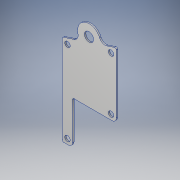
# Autodesk Inventor part: Column Plate
Saved by Autodesk Inventor 2019.4 (Build 234330000, 330)
## iProperties
Created: 2020-01-18
Part Number: Column Plate
Material: Aluminum 6061
Document SubType Name: Modeling
Designer: admin
Density: 2.7 g/cm^3
Appearance: Aluminum - Flat
Author: admin
Autodesk Inventor part; units mm, degrees
ref_plane "YZ Plane" through (0, 0, 0) normal (1, 0, 0) x (0, 1, 0)
ref_plane "XZ Plane" through (0, 0, 0) normal (0, 1, 0) x (-1, 0, 0)
ref_plane "XY Plane" through (0, 0, 0) normal (0, 0, 1) x (1, 0, 0)
sketch "Sketch1" plane through (0, 0, 0) normal (0, 0, 1) x (1, 0, 0)
  line L0 (0, 0) -> (-188.4, 0)
  line L1 (-188.4, 0) -> (-188.4, 316.0385)
  line L2 (-188.4, 316.0385) -> (0, 377.8495)
  circle A0 centre (-170.4, 303) radius 9.5
  circle A1 centre (-18, 353) radius 9.5
  circle A2 centre (-170.4, 18) radius 9.5
  circle A3 centre (-79, 86.5538) radius 88.9 construction
  line L3 (-188.4, 0) -> (-152.4, 0)
  line L4 (-152.4, 0) -> (-152.4, 150)
  line L5 (-152.4, 150) -> (0, 150)
  line L6 (0, 150) -> (0, 377.8495)
  circle A4 centre (-18, 168) radius 9.5
  circle A5 centre (-94.2, 287.3576) radius 88.9 construction
  circle A6 centre (-95, 363.5206) radius 16
  circle A7 centre (-95, 363.5206) radius 40
  dimension "d22" = 19
  dimension "d23" = 19
  dimension "d24" = 18
  dimension "d25" = 18
  dimension "d27" = 18
  dimension "d28" = 19
  dimension "d29" = 18
  dimension "d30" = 18
  dimension "d35" = 177.8
  dimension "d36" = 18
  dimension "d37" = 150
  dimension "d38" = 19
  dimension "d39" = 18
  dimension "d40" = 18
  dimension "d41" = 152.4
  dimension "d42" = 18
  dimension "d43" = 50
  dimension "d44" = 0
  dimension "d45" = 177.8
  dimension "d46" = 135
  dimension "d51" = 32
  dimension "d52" = 80
  dimension "d53" = 95
  constraints: 14 end point, 8 centre point, 2 point on line, 1 coincident, 1 horizontal, 1 parallel, 1 perpendicular, 1 tangent, 1 vertical
  measures "d22" diameter of A0
  measures "d23" diameter of A1
  measures "d24" distance from line of L1 A0.centre
  measures "d25" distance from line of L2 A0.centre
  measures "d27" distance from line of L2 A1.centre
  measures "d28" diameter of A2
  measures "d29" distance from line of L1 A2.centre
  measures "d30" distance from line of L0 A2.centre
  measures "d35" diameter of A3
  measures "d36" distance from line of L4 A2.centre
  measures "d37" distance of L3.end L4.end
  measures "d38" diameter of A4
  measures "d39" distance from line of L5 A4.centre
  measures "d40" distance from line of L6 A4.centre
  measures "d41" horizontal distance of A1.centre A0.centre
  measures "d42" distance from line of L6 A1.centre
  measures "d43" vertical distance of A1.centre A0.centre
  measures "d44" vertical distance of L4.end L5.end
  measures "d45" diameter of A5
  measures "d46" vertical distance of A4.centre A0.centre
  measures "d51" diameter of A6
  measures "d52" diameter of A7
  measures "d53" horizontal distance of L2.end A6.centre
extrude "Extrusion1" add sketch "Sketch1" along normal blind 5
fillet "Fillet1" radius 5 1 edges at (-188.4, 0, 2.5)
fillet "Fillet2" radius 15 2 edges at (-152.4, 0, 2.5) (0, 150, 2.5)
fillet "Fillet4" radius 5 2 edges at (-188.4, 316.0385, 2.5) (0, 377.8495, 2.5)
fillet "Fillet5" radius 20 2 edges at (-124.846, 336.8895, 2.5) (-55.1785, 359.7463, 2.5)
fillet "Fillet6" radius 5 1 edges at (-152.4, 150, 2.5)
body "Solid1"
